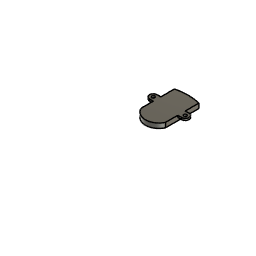
ProbeHolderAdaptor (Autodesk Fusion 360 design; units mm, degrees)
Autodesk Fusion 360 part; units mm, degrees
note: some values were not read from the file. Set by a fixed rule: which sketch regions a step uses.
sketch "Sketch1" plane through (0, 0, 140) normal (0, 0, -1) x (1, 0, 0)
  circle A0 centre (-34.641, -20) radius 6
  circle A1 centre (0, 40) radius 6
  circle A2 centre (34.641, -20) radius 6
  line L0 (-13.1, -15.8) -> (-20.5, -6.3321)
  line L1 (-21.6006, 6.5) -> (-21.6006, 7.5698)
  line L2 (-21.6006, 7.5698) -> (-12.2595, 14.2606)
  line L3 (-12.2595, 14.2606) -> (13.0954, 14.2606)
  line L4 (13.0954, 14.2606) -> (13.0954, -12.8135)
  line L5 (13.0954, -12.8135) -> (9.9759, -12.8135)
  arc A3 (9.9759, -12.8135) -> (-11.5482, -14.6776) centre (-0.0001, -22.8214) ccw
  line L6 (-11.5482, -14.6776) -> (-13.1, -15.8)
  line L7 (-38, 2.5) -> (-30, 2.5)
  line L8 (-30, 2.5) -> (-30, 6.5)
  line L9 (-30, 6.5) -> (-21.6006, 6.5)
  line L10 (-20.5, -6.5) -> (-30, -6.5)
  line L11 (-30, -6.5) -> (-30, -2.5)
  line L12 (-30, -2.5) -> (-38, -2.5)
  line L13 (-38, -2.5) -> (-38, 2.5)
  line L14 (20.5, -25.4) -> (20.5, -20.4)
  line L15 (20.5, -20.4) -> (28.5, -20.4)
  line L16 (28.5, -20.4) -> (28.5, -25.4)
  line L17 (28.5, -25.4) -> (20.5, -25.4)
  line L18 (20.5, 5.8) -> (20.5, 8.8)
  line L19 (20.5, 8.8) -> (28.5, 8.8)
  line L20 (28.5, 8.8) -> (28.5, 3.8)
  line L21 (28.5, 3.8) -> (22.5, 3.8)
  arc A4 (20.5, 5.8) -> (22.5, 3.8) centre (22.5, 5.8) ccw
  circle A5 centre (0, 0) radius 55
  line L22 (13, -58) -> (-13, -58)
  line L23 (-13, -58) -> (-13, -18)
  line L24 (-13, -18) -> (13, -18)
  line L25 (13, -18) -> (13, -58)
  line L26 (13, -58) -> (-13, -18) construction
  line L27 (-13, -58) -> (13, -18) construction
  line L28 (0, -38) -> (0, 0) construction
  arc A6 (13, -18) -> (-13, -18) centre (0, -24) ccw
  line L29 (-20.5, -6.3321) -> (-20.5, -6.5)
  point P0 (0, -38)
  dimension "d211" = 18
  dimension "d212" = 26
  dimension "d213" = 40
  dimension "d219" = 6
  constraint horizontal L22
  constraint perpendicular L22 L23
  constraint parallel L22 L24
  constraint parallel L23 L25
  constraint coincident L26 P0
  constraint coincident L27 P0
  constraint coincident P0 L28.start
  constraint vertical L28
  constraint coincident A5.centre L28.end
  measures "d211" distance of A5.centre L24
  measures "d212" distance of L23.end L24.end
  measures "d213" distance of L22.start L24.end
  measures "d219" distance of L24 A6.centre
extrude "Extrude1" add sketch "Sketch1" along normal blind 5 contours A5 L23 L24 L25 | L24 A6
sketch "Sketch3" plane through (0, 0, 135) normal (0, 0, -1) x (1, 0, 0)
  arc A0 (-13, -53.4416) -> (13, -53.4416) centre (0, 0) ccw
  line L0 (13, -53.4416) -> (13, -18)
  arc A1 (13, -18) -> (-13, -18) centre (0, -24) ccw
  line L1 (-13, -18) -> (-13, -53.4416)
  circle A2 centre (0, -18) radius 2.6
  line L2 (0, -18) -> (0, 0) construction
  line L3 (0, -15.4) -> (0, -20.6)
  dimension "d225" = 5.2
  dimension "d226" = 18
  constraint coincident A2.centre L2.start
  constraint coincident A0.centre L2.end
  constraint vertical L2
  constraint coincident A2 L3.start
  constraint coincident L2 L3.start
  constraint coincident A2 L3.end
  constraint parallel L2 L3
  measures "d225" diameter of A2
  measures "d226" distance of A2.centre A0.centre
revolve "Revolve1" cut sketch "Sketch3" angle 360 about axis through (0, 15.4, 135) along (0, 1, 0) contours A2 L3 picked at (0.8578, -17.8767)
sketch "Sketch6" plane through (0, 0, 140) normal (0, 0, 1) x (-1, 0, 0)
  arc A0 (-13, -53.4416) -> (13, -53.4416) centre (0, 0) ccw
  line L0 (13, -53.4416) -> (13, -18)
  arc A1 (13, -18) -> (-13, -18) centre (0, -24) ccw
  line L1 (-13, -18) -> (-13, -53.4416)
  circle A2 centre (17, -35) radius 1.6
  circle A3 centre (17, -35) radius 4
  line L2 (17, -31) -> (13, -31)
  line L3 (13, -31) -> (13, -39)
  line L4 (13, -39) -> (17, -39)
  line L5 (17, -39) -> (17, -31)
  line L6 (0, -9.6822) -> (0, -55) construction
  line L7 (-17, -31) -> (-13, -31)
  line L8 (-13, -39) -> (-17, -39)
  circle A4 centre (-17, -35) radius 4
  circle A5 centre (-17, -35) radius 1.6
  dimension "d228" = 3.2
  dimension "d229" = 8
  dimension "d230" = 35
  dimension "d231" = 4
  constraint concentric A2 A3
  constraint horizontal L2
  constraint vertical L3
  constraint horizontal L4
  constraint vertical L5
  constraint coincident L0 L3.end
  constraint coincident A3 L2.start
  constraint tangent A3 L4
  constraint tangent A3 L2
  constraint midpoint A1 L6.start
  constraint midpoint A0 L6.end
  constraint symmetric A2 L6 A5
  constraint symmetric A3 L6 A4
  constraint symmetric L2.start L6 L7.start
  constraint symmetric L2.end L6 L7.end
  constraint symmetric L3.end L6 L8.start
  constraint symmetric L4.end L6 L8.end
  measures "d228" diameter of A2
  measures "d229" diameter of A3
  measures "d230" vertical distance of A0.centre A2.centre
  measures "d231" distance of L0 A2.centre
extrude "Extrude2" add sketch "Sketch6" against normal blind 2 contours L1 L8 A4 | L0 A3 L3 L4 | L1 L7 A4 | A4 | L0 A3 L2 L3 | A2 A3 L5 | A2 A3 L5
sketch "Sketch9" plane through (0, 0, 135) normal (0, 0, -1) x (1, 0, 0)
  circle A0 centre (0, -18) radius 2.6
  arc A1 (-13, -53.4416) -> (13, -53.4416) centre (0, 0) ccw
  line L0 (13, -53.4416) -> (13, -18)
  arc A2 (13, -18) -> (-13, -18) centre (0, -24) ccw
  line L1 (-13, -18) -> (-13, -53.4416)
  line L2 (13, -23) -> (13, -38)
  line L3 (-13, -38) -> (-13, -23)
  circle A3 centre (0, -30) radius 3.05
  circle A4 centre (0, -38) radius 3.05
  line L4 (0, -30) -> (0, -38) construction
  circle A5 centre (-8, -30) radius 3.05
  circle A6 centre (-8, -38) radius 3.05
  circle A7 centre (8, -30) radius 3.05
  circle A8 centre (8, -38) radius 3.05
  dimension "d302" = 6.1
  dimension "d303" = 6.1
  dimension "d304" = 8
  dimension "d305" = 12
  dimension "d308" = 8
  dimension "d309" = 0
  constraint vertical L2
  constraint vertical L3
  constraint coincident L0 L2.end
  constraint coincident L1 L3.end
  constraint coincident A3.centre L4.start
  constraint coincident A4.centre L4.end
  constraint vertical L4
  constraint coincident A0.centre L4
  measures "d302" diameter of A3
  measures "d303" diameter of A4
  measures "d304" distance of A3.centre A4.centre
  measures "d305" distance of A0.centre A3.centre
extrude "Extrude5" cut sketch "Sketch9" against normal blind 2.1 contours A0 | A3 | A4 | A5 | A6 | A7 | A8
